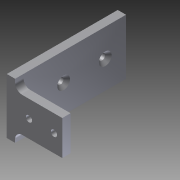
# Autodesk Inventor part: 1_0204_003
Saved by Autodesk Inventor 2012 SP1 (Build 160190100, 190)
## iProperties
Created: 2013-03-21
Part Number: 1_0204_003
Material: Default
Document SubType Name: Modeling
Designer: vogel
Density: 1 g/cm^3
Author: vogel
Autodesk Inventor part; units mm, degrees
ref_plane "YZ Plane" through (0, 0, 0) normal (1, 0, 0) x (0, 1, 0)
ref_plane "XZ Plane" through (0, 0, 0) normal (0, 1, 0) x (-1, 0, 0)
ref_plane "XY Plane" through (0, 0, 0) normal (0, 0, 1) x (1, 0, 0)
sketch "Skizze1" plane through (0, 0, 0) normal (0, 0, 1) x (1, 0, 0)
  line L0 (0, 0) -> (2.7641, 0)
  line L1 (6, 6) -> (6, 80)
  line L2 (6, 80) -> (0, 80)
  line L3 (0, 80) -> (0, 0)
  line L4 (-8, 0) -> (48, 0) projected
  line L5 (0, -16) -> (0, 96) projected
  line L6 (0, 0) -> (40, 0)
  line L7 (40, 0) -> (40, 6)
  line L8 (40, 6) -> (6, 6)
  line L9 (0, 2.8256) -> (0, 0)
  dimension "d0" = 80
  dimension "d1" = 40
  dimension "d2" = 6
  constraints: 16 end point, 4 parallel, 3 perpendicular, 2 horizontal
  measures "d0" distance of L2.end L0.start
  measures "d1" distance of L0.start L6.end
  measures "d2" distance between parallel lines of L8 L6
extrude "Extrusion1" add sketch "Skizze1" along normal blind 40
sketch "Skizze2" plane through (6, 6, 0) normal (0, 1, 0) x (1, 0, 0)
  line L0 (34, 0) -> (34, -40) projected
  line L1 (0, 0) -> (0, -40) projected
  line L2 (0, -20) -> (34, -20)
  line L3 (0, -7.5) -> (34, -7.5)
  line L4 (34, -7.5) -> (34, -32.5)
  line L5 (34, -32.5) -> (0, -32.5)
  line L6 (0, -32.5) -> (0, -7.5)
  line L7 (34, -7.5) -> (0, -7.5)
  line L8 (0, -7.5) -> (0, 0)
  line L9 (0, 0) -> (34, 0)
  line L10 (34, 0) -> (34, -7.5)
  line L11 (34, -40) -> (0, -40)
  line L12 (0, -40) -> (0, -32.5)
  line L13 (0, -32.5) -> (34, -32.5)
  line L14 (34, -32.5) -> (34, -40)
  point P0 (-6, 0)
  dimension "d5" = 25
  constraints: 26 end point, 6 parallel, 3 horizontal, 3 perpendicular, 2 midpoint, 2 point on line, 1 other
  measures "d5" distance between parallel lines of L5 L3
extrude "Extrusion2" cut sketch "Skizze2" against normal through all contours L0 L3 L1 L9 | L0 L11 L1 L5
sketch "Skizze3" plane through (0, 0, 0) normal (-1, 0, 0) x (0, 0, 1)
  line L0 (0, 80) -> (40, 80) projected
  line L1 (0, 0) -> (40, 0) projected
  line L2 (20, 80) -> (20, 0)
  point P0 (20, 65)
  point P1 (20, 35)
  dimension "d8" = 15
  dimension "d9" = 30
  constraints: 2 end point, 2 midpoint, 2 point on line
  measures "d8" distance from line of point (20, 65) L0
  measures "d9" distance of point (20, 35) point (20, 65)
hole "Bohrung1" at (0, 65, 20) at (0, 35, 20) direction (1, 0, 0) diameter 4 end through all
sketch "Skizze4" plane through (6, 6, 32.5) normal (0, 1, 0) x (1, 0, 0)
  line L0 (34, 25) -> (34, 0) projected
  line L1 (0, 25) -> (0, 0) projected
  line L2 (34, 12.5) -> (0, 12.5)
  point P0 (-6, 32.5)
  point P1 (28, 12.5)
  point P2 (10, 12.5)
  dimension "d17" = 18
  dimension "d44" = 6
  constraints: 2 end point, 2 midpoint, 2 point on line
  measures "d17" distance of point (28, 12.5) point (10, 12.5)
  measures "d44" distance from line of L0 point (28, 12.5)
hole "Bohrung2" at (34, 6, 20) at (16, 6, 20) direction (0, -1, 0) diameter 4.5 end through all
fillet "Rundung1" radius 5 2 edges at (6, 3, 32.5) (6, 3, 7.5)
sketch "Skizze5" plane through (6, 0, 0) normal (1, 0, 0) x (0, 0, -1)
  circle A0 centre (-20, 65) radius 2 projected
  circle A1 centre (-20, 35) radius 2 projected
  constraints: 2 coincident
hole "Bohrung5" at (6, 65, 20) at (6, 35, 20) direction (-1, 0, 0) diameter 4.5 end through all countersink diameter 9.2 countersink angle 90
